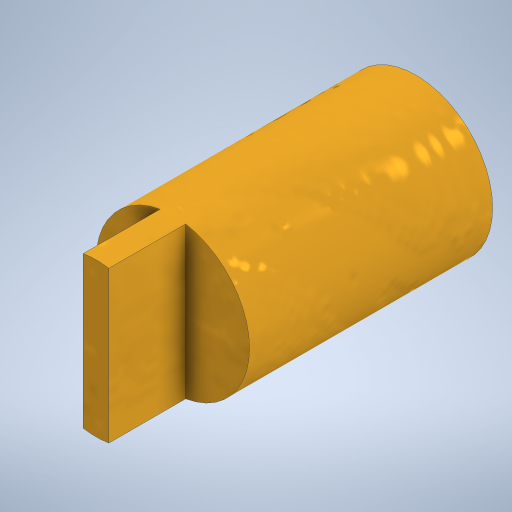
# Autodesk Inventor part: Лазер маленький
Saved by Autodesk Inventor 2024 (Build 280153020, 153B)
## iProperties
Created: 2022-11-06
Part Number: Лазер маленький
Material: Типовые
Document SubType Name: Modeling
Designer: Admin
Density: 1 g/cm^3
Appearance: По умолчанию
Author: Admin
Autodesk Inventor part; units mm, degrees
ref_plane "YZ Plane" through (0, 0, 0) normal (1, 0, 0) x (0, 1, 0)
ref_plane "XZ Plane" through (0, 0, 0) normal (0, 1, 0) x (-1, 0, 0)
ref_plane "XY Plane" through (0, 0, 0) normal (0, 0, 1) x (1, 0, 0)
sketch "Эскиз1" plane through (0, 0, 0) normal (0, 0, 1) x (1, 0, 0)
  circle A0 centre (0, 0) radius 3
  dimension "d0" = 6
  constraints: 1 centre point, 1 coincident
  measures "d0" diameter of A0
extrude "Выдавливание1" add sketch "Эскиз1" along normal blind 9.5
sketch "Эскиз2" plane through (0, 0, 9.5) normal (0, 0, 1) x (1, 0, 0)
  circle A0 centre (0, 0) radius 3 projected
  line L0 (-0.5, 2.958) -> (-0.5, -2.958)
  line L1 (0.5, -2.958) -> (0.5, 2.958)
  line L2 (0, 0) -> (0, 0.4981) construction
  dimension "d3" = 1
  constraints: 6 end point, 4 point on circle, 2 vertical, 1 parallel, 1 other
  measures "d3" distance between parallel lines of L0 L1
extrude "Выдавливание2" add sketch "Эскиз2" along normal blind 3 contours L1 A0 L0
sketch "Эскиз3" plane through (0, 0, 0) normal (0, 0, -1) x (-1, 0, 0)
  circle A0 centre (0, 0) radius 2
  dimension "d6" = 4
  constraints: 1 centre point, 1 coincident
  measures "d6" diameter of A0
extrude "Выдавливание3" cut sketch "Эскиз3" against normal blind 2
sketch "Эскиз4" plane through (0, 0, 2) normal (0, 0, -1) x (-1, 0, 0)
  circle A0 centre (0, 0) radius 2 projected
extrude "Выдавливание4" add sketch "Эскиз4" along normal blind 100 separate body
